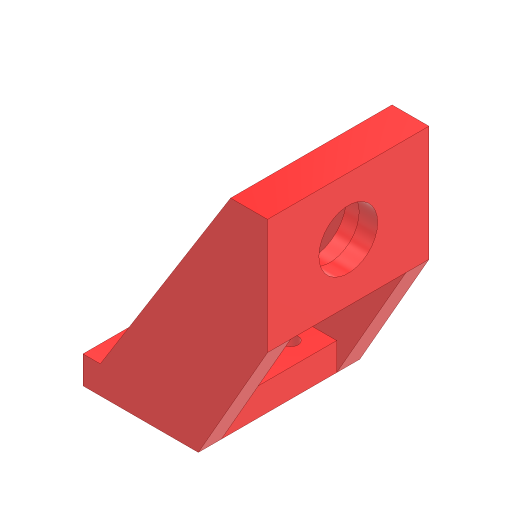
# Autodesk Inventor part: Part15
Saved by Autodesk Inventor 2024.3 (Build 283343000, 343)
## iProperties
Created: 2025-06-09
Part Number: Part15
Material: Generic
Document SubType Name: Modeling
Designer: MPA
Density: 1 g/cm^3
Appearance: Light Red
Author: MPA
## iProperties of the stored document Part15_3DPrint.ipt
Created: 2025-06-18
Part Number: Part15_3DPrint
Material: Generic
Document SubType Name: Modeling
Designer: MPA
Density: 1 g/cm^3
Appearance: Default
Author: MPA
Autodesk Inventor part; units mm, degrees
ref_plane "YZ Plane" through (0, 0, 0) normal (1, 0, 0) x (0, 1, 0)
ref_plane "XZ Plane" through (0, 0, 0) normal (0, 1, 0) x (-1, 0, 0)
ref_plane "XY Plane" through (0, 0, 0) normal (0, 0, 1) x (1, 0, 0)
sketch "Sketch1" plane through (0, 0, 0) normal (1, 0, 0) x (0, 1, 0)
  line L0 (-25, 35) -> (25, 35)
  line L1 (25, 35) -> (25, -35)
  line L2 (25, -35) -> (-25, -35)
  line L3 (-25, -35) -> (-25, 35)
  line L4 (-25, 35) -> (25, -35) construction
  line L5 (25, 35) -> (-25, -35) construction
  point P0 (0, 0)
  dimension "d0" = 50
  dimension "d1" = 70
  constraints: 12 end point, 2 midpoint, 2 parallel, 1 horizontal, 1 perpendicular
  measures "d0" distance of L1.end L2.end
  measures "d1" distance of L0.end L1.end
extrude "Extrusion1" add sketch "Sketch1" along normal blind 16
sketch "Sketch2" plane through (16, 0, 0) normal (1, 0, 0) x (0, 0, -1)
  circle A0 centre (0, 0) radius 15.25
  dimension "d4" = 30.5
  constraints: 1 centre point, 1 coincident
  measures "d4" diameter of A0
extrude "Extrusion2" cut sketch "Sketch2" against normal through all
sketch "Sketch3" plane through (16, 0, 0) normal (1, 0, 0) x (0, 0, -1)
  circle A0 centre (0, 0) radius 15.25 projected
  circle A1 centre (0, 0) radius 12.75
  dimension "d7" = 25.5
  constraints: 1 centre point, 1 coincident
  measures "d7" diameter of A1
extrude "Extrusion3" add sketch "Sketch3" against normal blind 8
sketch "Sketch4" plane through (0, -25, 35) normal (0, 0, 1) x (1, 0, 0)
  line L0 (0, 50) -> (0, 0) projected
  line L1 (0, 0) -> (16, 0) projected
  line L2 (16, 50) -> (16, 0) projected
  line L3 (0, 50) -> (16, 50) projected
  line L4 (16, 37.75) -> (16, 12.25) projected
  line L5 (8, 12.25) -> (8, 37.75) projected
  line L6 (16, 37.75) -> (16, 12.25) projected
  line L7 (16, 50) -> (-64, 50)
  line L8 (-64, 50) -> (-64, -52.5)
  line L9 (-64, -52.5) -> (16, -52.5)
  line L10 (16, -52.5) -> (16, 50)
  line L11 (0, 50) -> (-64, -52.5)
  line L12 (16, 0) -> (-14, -52.5)
  point P0 (0, 25)
  point P1 (8, 25)
  dimension "d10" = 77.5
  dimension "d11" = 80
  dimension "d12" = 50
  constraints: 12 end point, 2 parallel, 1 horizontal, 1 midpoint, 1 perpendicular, 1 point on line
  measures "d10" distance from line of point (8, 25) L9
  measures "d11" distance of L2.start L7.end
  measures "d12" distance of L8.end L12.end
extrude "Extrusion4" add sketch "Sketch4" against normal blind 10 contours L0 L1 L12 L9 L11
mirror "Mirror1" about plane through (0, 0, 0) normal (0, 0, 1) of "Extrusion4"
sketch "Sketch5" plane through (-64, -77.5, 35) normal (0, -1, 0) x (1, 0, 0)
  line L0 (0, 0) -> (50, 0) projected
  line L1 (0, 0) -> (0, -10) projected
  line L2 (50, -10) -> (0, -10) projected
  line L3 (50, 0) -> (50, -10) projected
  line L4 (0, -70) -> (50, -70) projected
  line L5 (50, -70) -> (50, -60) projected
  line L6 (50, -60) -> (0, -60) projected
  line L7 (0, -70) -> (0, -60) projected
  line L8 (0, 0) -> (50, 0)
  line L9 (50, 0) -> (50, -70)
  line L10 (50, -70) -> (0, -70)
  line L11 (0, -70) -> (0, 0)
  point P0 (64, -35)
  constraints: 8 end point, 2 parallel, 1 horizontal, 1 perpendicular
extrude "Extrusion5" add sketch "Sketch5" against normal blind 12
sketch "Sketch6" plane through (-64, -65.5, 35) normal (0, 1, 0) x (1, 0, 0)
  line L0 (50, 10) -> (7.4927, 10) projected
  line L1 (50, 10) -> (50, 60) projected
  line L2 (7.4927, 60) -> (50, 60) projected
  line L3 (7.4927, 70) -> (7.4927, 60) projected
  line L4 (7.4927, 70) -> (0, 70) projected
  line L5 (0, 70) -> (0, 0) projected
  line L6 (0, 0) -> (7.4927, 0) projected
  line L7 (7.4927, 10) -> (7.4927, 0) projected
  line L8 (64, 70) -> (7.4927, 70) projected
  line L9 (64, 70) -> (80, 70) projected
  line L10 (50, 70) -> (80, 70) projected
  line L11 (0, 70) -> (50, 70) projected
  line L12 (7.4927, 70) -> (0, 70) projected
  line L13 (50, 0) -> (80, 0) projected
  line L14 (64, 0) -> (80, 0) projected
  line L15 (64, 0) -> (7.4927, 0) projected
  line L16 (0, 0) -> (7.4927, 0) projected
  line L17 (0, 0) -> (50, 0) projected
  line L18 (50, 0) -> (0, 70) construction
  line L19 (50, 70) -> (0, 0) construction
  line L20 (10, 20) -> (40, 20) construction
  line L21 (40, 20) -> (40, 50) construction
  line L22 (40, 50) -> (10, 50) construction
  line L23 (10, 50) -> (10, 20) construction
  line L24 (10, 20) -> (40, 50) construction
  line L25 (40, 20) -> (10, 50) construction
  point P0 (64, 35)
  point P1 (25, 35)
  dimension "d17" = 30
  dimension "d18" = 30
  constraints: 16 end point, 4 coincident, 4 point on line, 3 midpoint, 2 parallel, 1 horizontal, 1 perpendicular
  measures "d17" distance of L22.end L21.end
  measures "d18" distance of L21.end L20.end
hole "Hole1" at (-24, -65.5, -15) at (-54, -65.5, -15) at (-54, -65.5, 15) at (-24, -65.5, 15) direction (0, -1, 0) diameter 6.6 end through all clearance for "Countersunk Flat Head Screw DIN EN ISO 2009" size "M6" standard "DIN"
body "Solid1"
